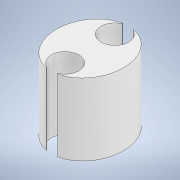
# Autodesk Inventor part: Relleno_chumacera
Saved by Autodesk Inventor 2020 (Build 240168000, 168)
## iProperties
Created: 2021-01-14
Part Number: Relleno_chumacera
Material: Plástico PC/ABS
Document SubType Name: Modeling
Designer: Cerberus 1S
Density: 0.357273 g/cm^3
Appearance: Suave - Blanco
Author: Cerberus 1S
Autodesk Inventor part; units mm, degrees
ref_plane "YZ Plane" through (0, 0, 0) normal (1, 0, 0) x (0, 1, 0)
ref_plane "XZ Plane" through (0, 0, 0) normal (0, 1, 0) x (-1, 0, 0)
ref_plane "XY Plane" through (0, 0, 0) normal (0, 0, 1) x (1, 0, 0)
sketch "Boceto1" plane through (0, 0, 0) normal (0, 1, 0) x (-1, 0, 0)
  ellipse E0 centre (0, 0) end of major axis (0, 7) minor radius 6.05
  circle A0 centre (0, -4.5) radius 2.5
  circle A1 centre (0, 4.5) radius 2.5
  point P0 (0, 7)
  point P1 (0, -7)
  dimension "d0" = 7
  dimension "d1" = 6.05
  dimension "d6" = 5
  dimension "d7" = 5
  constraints: 2 centre point, 2 vertical alignment, 1 coincident, 4 other
  measures "d6" diameter of A0
  measures "d7" diameter of A1
extrude "Extrusión1" add sketch "Boceto1" along normal blind 13
sketch "Boceto2" plane through (0, 13, 4.5) normal (0, 1, 0) x (1, 0, 0)
  line L0 (-1, -2) -> (1, -2)
  line L1 (1, -2) -> (1, -4)
  line L2 (1, -4) -> (-1, -4)
  line L3 (-1, -4) -> (-1, -2)
  circle A0 centre (0, 0) radius 2.5 projected
  point P0 (0, 4.5)
  point P1 (0, -2.5)
  dimension "d8" = 2
  dimension "d9" = 1
  dimension "d11" = 2
  dimension "d12" = 2
  constraints: 8 end point, 2 parallel, 1 horizontal, 1 perpendicular, 1 vertical alignment
  measures "d8" distance from line of point (0, 0) L0
  measures "d9" distance from line of point (0, 0) L3
  measures "d11" distance between parallel lines of L2 L0
  measures "d12" distance between parallel lines of L1 L3
extrude "Extrusión2" cut sketch "Boceto2" against normal blind 13 contours L0 L1 A0 L3 | A0 L1 L2 L3 picked at (0, -2.1667)
sketch "Boceto4" plane through (0, 13, 0) normal (0, 1, 0) x (1, 0, 0)
  line L0 (-1, 8) -> (1, 8)
  line L1 (1, 8) -> (1, 4.3137)
  line L2 (1, 4.3137) -> (-1, 4.3137)
  line L3 (-1, 4.3137) -> (-1, 8)
  point P0 (0, 0)
  dimension "d15" = 2
  dimension "d16" = 4.3137
  dimension "d17" = 8
  dimension "d18" = 1
  constraints: 8 end point, 2 parallel, 1 horizontal, 1 perpendicular
  measures "d15" distance between parallel lines of L1 L3
  measures "d16" distance from line of point (0, 0) L2
  measures "d17" distance from line of point (0, 0) L0
  measures "d18" distance from line of point (0, 0) L3
extrude "Extrusión3" cut sketch "Boceto4" against normal blind 13
equation "\"d7\" = d6"
equation "\"d9\" = 0.5 * d12"
equation "\"d18\" = 0.5 * d15"
